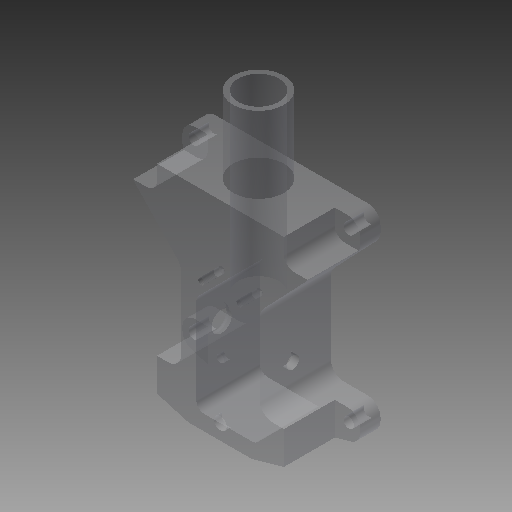
# Autodesk Inventor part: LCD Olfaktometerkammer
Saved by Autodesk Inventor 2018 (Build 220112000, 112)
## iProperties
Created: 2010-08-23
Part Number: LCD Olfaktometerkammer
Document SubType Name: Modeling
Designer: neef
Density: 1 g/cm^3
Material: Generic
Appearance: Polycarbonate - Clear
Author: neef
Autodesk Inventor part; units mm, degrees
ref_plane "YZ Plane" through (0, 0, 0) normal (1, 0, 0) x (0, 1, 0)
ref_plane "XZ Plane" through (0, 0, 0) normal (0, 1, 0) x (-1, 0, 0)
ref_plane "XY Plane" through (0, 0, 0) normal (0, 0, 1) x (1, 0, 0)
sketch "Skizze1" plane through (0, 0, 0) normal (0, 0, 1) x (1, 0, 0)
  line L0 (-3.4427, -24.7647) -> (-3.4427, -50.7647) projected
  line L1 (-3.4427, -50.7647) -> (-23.4427, -50.7647) projected
  line L2 (-23.4427, -50.7647) -> (-23.4427, -24.7647) projected
  line L3 (-23.4427, -24.7647) -> (-3.4427, -24.7647) projected
  circle A0 centre (-43.9427, -51.2647) radius 2.1 projected
  circle A1 centre (17.0573, -51.2647) radius 2.1 projected
  circle A2 centre (17.0573, 14.7353) radius 2.1 projected
  circle A3 centre (-43.9427, 14.7353) radius 2.1 projected
  line L4 (21.5573, 19.2353) -> (21.5573, -55.7647) projected
  line L5 (-48.4427, 19.2353) -> (21.5573, 19.2353) projected
  line L6 (-48.4427, -55.7647) -> (-48.4427, 19.2353) projected
  line L7 (21.5573, -55.7647) -> (-48.4427, -55.7647) projected
  line L8 (-48.4427, 19.2353) -> (21.5573, 19.2353)
  line L9 (21.5573, 19.2353) -> (21.5573, -55.7647)
  line L10 (-48.4427, -55.7647) -> (-48.4427, 19.2353)
  line L11 (0, 37.2353) -> (0, -88.7647) projected
  line L12 (-62.4427, 0) -> (35.5573, 0) projected
  line L13 (-48.4427, -55.7647) -> (-48.4427, -70.7647)
  line L14 (-48.4427, -70.7647) -> (21.5573, -70.7647)
  line L15 (21.5573, -70.7647) -> (21.5573, -55.7647)
  dimension "d9" = 15
  constraints: 12 end point, 3 perpendicular, 2 parallel, 1 horizontal
  measures "d9" distance between parallel lines of L7 L14
extrude "Extrusion1" add sketch "Skizze1" along normal blind 28 contours L0 L1 L2 L3 | A0 | A1 | A2 | A3 | L4 L12 L11 L5 | L4 L7 L11 L12 | L11 L12 L6 L5 | L15 L14 L11 L7 | L11 L7 L6 L12 | L11 L14 L13 L7
sketch "Skizze2" plane through (0, 0, 0) normal (0, 0, -1) x (-1, 0, 0)
  line L0 (-21.5573, -70.7647) -> (-21.5573, 19.2353) projected
  line L1 (0.9427, -19.7647) -> (25.9427, -19.7647)
  line L2 (25.9427, -19.7647) -> (25.9427, -59.7647)
  line L3 (25.9427, -59.7647) -> (0.9427, -59.7647)
  line L4 (0.9427, -59.7647) -> (0.9427, -19.7647)
  line L5 (3.4427, -50.7647) -> (3.4427, -24.7647) projected
  line L6 (48.4427, 19.2353) -> (48.4427, -70.7647) projected
  line L7 (-21.5573, 19.2353) -> (48.4427, 19.2353) projected
  line L8 (-21.5573, -70.7647) -> (-21.5573, 19.2353) projected
  line L9 (3.4427, -24.7647) -> (23.4427, -24.7647) projected
  line L10 (23.4427, -24.7647) -> (23.4427, -50.7647) projected
  line L11 (23.4427, -50.7647) -> (3.4427, -50.7647) projected
  line L12 (48.4427, -70.7647) -> (-21.5573, -70.7647) projected
  point P0 (-21.5573, -55.7647)
  dimension "d2" = 25
  dimension "d3" = 40
  dimension "d5" = 22.5
  dimension "d6" = 5
  constraints: 8 end point, 2 parallel, 1 horizontal, 1 perpendicular
  measures "d2" distance of L2.end L3.end
  measures "d3" distance of L1.end L2.end
  measures "d5" distance between parallel lines of L4 L0
  measures "d6" distance between parallel lines of L9 L1
extrude "Extrusion2" cut sketch "Skizze2" against normal blind 25 contours L1 L2 L3 L4 | L5 L9 L10 L11
sketch "Skizze3" plane through (-48.4427, 19.2353, 0) normal (0, 1, 0) x (1, 0, 0)
  line L0 (0, -28) -> (70, -28) projected
  line L1 (70, 0) -> (70, -28) projected
  circle A0 centre (35, -13) radius 10
  circle A1 centre (35, -13) radius 8
  dimension "d10" = 16
  dimension "d11" = 20
  dimension "d12" = 15
  dimension "d13" = 35
  constraints: 2 centre point, 1 coincident
  measures "d10" diameter of A1
  measures "d11" diameter of A0
  measures "d12" distance from line of L0 A1.centre
  measures "d13" distance from line of L1 A1.centre
extrude "Extrusion3" add sketch "Skizze3" along normal blind 30
sketch "Skizze4" plane through (-13.4427, 19.2353, 13) normal (0, 1, 0) x (1, 0, 0)
  circle A0 centre (0, 0) radius 8 projected
  circle A1 centre (0, 0) radius 8 projected
  circle A2 centre (0, 0) radius 8
  constraints: 1 centre point, 1 coincident, 1 concentric
extrude "Extrusion4" cut sketch "Skizze4" against normal up to surface (39 mm away)
fillet "Rundung1" radius 3 4 edges at (-0.9427, -19.7647, 12.5) (-25.9427, -19.7647, 12.5) (-0.9427, -59.7647, 12.5) (-25.9427, -59.7647, 12.5)
sketch "Skizze5" plane through (0, 0, 28) normal (0, 0, 1) x (1, 0, 0)
  circle A0 centre (-43.9427, 14.7353) radius 2.1 projected
  circle A1 centre (17.0573, 14.7353) radius 2.1 projected
  circle A2 centre (17.0573, -51.2647) radius 2.1 projected
  circle A3 centre (-43.9427, -51.2647) radius 2.1 projected
extrude "Extrusion5" cut sketch "Skizze5" against normal up to surface (28 mm away)
sketch "Skizze6" plane through (0, 0, 25) normal (0, 0, -1) x (-1, 0, 0)
  line L0 (25.9427, -56.7647) -> (25.9427, -22.7647) projected
  line L1 (22.9427, -19.7647) -> (3.9427, -19.7647) projected
  circle A0 centre (13.4427, -34.7647) radius 1.5
  line L2 (3.9427, -59.7647) -> (22.9427, -59.7647) projected
  circle A1 centre (13.4427, -56.7647) radius 2.5
  dimension "d21" = 3
  dimension "d22" = 15
  dimension "d23" = 12.5
  dimension "d58" = 5
  dimension "d59" = 12.5
  dimension "d60" = 3
  constraints: 2 centre point
  measures "d21" diameter of A0
  measures "d22" distance from line of L1 A0.centre
  measures "d23" distance from line of L0 A0.centre
  measures "d58" diameter of A1
  measures "d59" distance from line of L0 A1.centre
  measures "d60" distance from line of L2 A1.centre
extrude "Extrusion6" cut sketch "Skizze6" against normal up to surface (3 mm away)
sketch "Skizze7" plane through (21.5573, -70.7647, 0) normal (1, 0, 0) x (0, 0, -1)
  circle A0 centre (-15, 36) radius 2.45
  line L0 (-25, 37.5) -> (-28, 37.5) projected
  line L1 (-25, 34.5) -> (-28, 34.5) projected
  line L2 (-25, 48) -> (-25, 14) projected
  line L3 (0, 48) -> (-25, 48) projected
  dimension "d26" = 1.5
  dimension "d27" = 4.9
  dimension "d28" = 10
  constraints: 1 centre point
  measures "d26" distance from line of A0.centre L1
  measures "d27" diameter of A0
  measures "d28" distance from line of L2 A0.centre
extrude "Extrusion7" cut sketch "Skizze7" against normal up to surface (70 mm away)
sketch "Skizze8" plane through (0, 0, 0) normal (0, 0, -1) x (-1, 0, 0)
  circle A0 centre (43.9427, -51.2647) radius 2.1 projected
  circle A1 centre (43.9427, 14.7353) radius 2.1 projected
  circle A2 centre (-17.0573, 14.7353) radius 2.1 projected
  circle A3 centre (-17.0573, -51.2647) radius 2.1 projected
  line L0 (0.9427, -56.7647) -> (0.9427, -22.7647) projected
  arc A4 (3.9427, -19.7647) -> (0.9427, -22.7647) centre (3.9427, -22.7647) ccw projected
  line L1 (3.9427, -19.7647) -> (22.9427, -19.7647) projected
  arc A5 (25.9427, -22.7647) -> (22.9427, -19.7647) centre (22.9427, -22.7647) ccw projected
  line L2 (25.9427, -22.7647) -> (25.9427, -56.7647) projected
  arc A6 (22.9427, -59.7647) -> (25.9427, -56.7647) centre (22.9427, -56.7647) ccw projected
  line L3 (22.9427, -59.7647) -> (3.9427, -59.7647) projected
  arc A7 (0.9427, -56.7647) -> (3.9427, -59.7647) centre (3.9427, -56.7647) ccw projected
  line L4 (48.4427, 19.2353) -> (48.4427, -70.7647) projected
  line L5 (-21.5573, 19.2353) -> (48.4427, 19.2353) projected
  line L6 (-21.5573, -70.7647) -> (-21.5573, 19.2353) projected
  line L7 (48.4427, -70.7647) -> (-21.5573, -70.7647) projected
  line L8 (13.4427, -79.9912) -> (13.4427, -69.4061)
  line L9 (48.4427, -70.7647) -> (-21.5573, -70.7647) projected
  line L10 (13.4427, -69.4061) -> (13.4427, 58.2519)
  line L11 (-21.5573, 19.2353) -> (48.4427, 19.2353) projected
  line L12 (13.4427, 19.2353) -> (-16.5573, 19.2353)
  line L13 (-21.5573, 19.2353) -> (-21.5573, 9.7353)
  line L14 (-21.5573, 19.2353) -> (-21.5573, -70.7647) projected
  line L15 (-20.18, 8.2875) -> (-3.4345, -9.3169)
  line L16 (-2.0573, -12.7629) -> (-2.0573, -41.2647)
  line L17 (-7.0573, -46.2647) -> (-16.5573, -46.2647)
  line L18 (-21.5573, 11.7335) -> (-21.5573, 14.2353)
  line L19 (-21.5573, -46.2647) -> (-21.5573, 19.2353)
  line L20 (13.4427, -62.7647) -> (1.6505, -62.7647)
  line L21 (0.2628, -62.5683) -> (-17.9449, -57.3083)
  line L22 (-21.5573, -52.5047) -> (-21.5573, -51.2647)
  arc A8 (-16.5573, 19.2353) -> (-21.5573, 14.2353) centre (-16.5573, 14.2353) ccw
  arc A9 (-21.5573, 11.7335) -> (-20.18, 8.2875) centre (-16.5573, 11.7335) ccw
  arc A10 (-2.0573, -12.7629) -> (-3.4345, -9.3169) centre (-7.0573, -12.7629) ccw
  arc A11 (-7.0573, -46.2647) -> (-2.0573, -41.2647) centre (-7.0573, -41.2647) ccw
  arc A12 (-16.5573, -46.2647) -> (-21.5573, -51.2647) centre (-16.5573, -51.2647) ccw
  arc A13 (-21.5573, -52.5047) -> (-17.9449, -57.3083) centre (-16.5573, -52.5047) ccw
  arc A14 (0.2628, -62.5683) -> (1.6505, -62.7647) centre (1.6505, -57.7647) ccw
  circle A15 centre (43.9427, 14.7353) radius 2.1
  circle A16 centre (43.9427, -51.2647) radius 2.1
  line L23 (48.4427, -70.7647) -> (48.4427, 19.2353)
  line L24 (13.4427, 19.2353) -> (43.4427, 19.2353)
  line L25 (48.4427, 19.2353) -> (48.4427, 9.7353)
  line L26 (47.0655, 8.2875) -> (30.32, -9.3169)
  line L27 (28.9427, -12.7629) -> (28.9427, -41.2647)
  line L28 (33.9427, -46.2647) -> (43.4427, -46.2647)
  line L29 (48.4427, 11.7335) -> (48.4427, 14.2353)
  line L30 (13.4427, -62.7647) -> (25.235, -62.7647)
  line L31 (26.6227, -62.5683) -> (44.8304, -57.3083)
  line L32 (48.4427, -52.5047) -> (48.4427, -51.2647)
  arc A17 (48.4427, 14.2353) -> (43.4427, 19.2353) centre (43.4427, 14.2353) ccw
  arc A18 (47.0655, 8.2875) -> (48.4427, 11.7335) centre (43.4427, 11.7335) ccw
  arc A19 (30.32, -9.3169) -> (28.9427, -12.7629) centre (33.9427, -12.7629) ccw
  arc A20 (28.9427, -41.2647) -> (33.9427, -46.2647) centre (33.9427, -41.2647) ccw
  arc A21 (48.4427, -51.2647) -> (43.4427, -46.2647) centre (43.4427, -51.2647) ccw
  arc A22 (44.8304, -57.3083) -> (48.4427, -52.5047) centre (43.4427, -52.5047) ccw
  arc A23 (25.235, -62.7647) -> (26.6227, -62.5683) centre (25.235, -57.7647) ccw
  point P0 (-2.0573, -10.7647)
  point P1 (0.9427, -62.7647)
  point P2 (-21.5573, -56.2647)
  point P3 (28.9427, -10.7647)
  point P4 (48.4427, -46.2647)
  point P5 (25.9427, -62.7647)
  point P6 (48.4427, -56.2647)
  dimension "d47" = 0
  dimension "d48" = 3
  dimension "d49" = 35
  dimension "d50" = 5
  dimension "d51" = 5
  dimension "d52" = 3
  dimension "d53" = 30
  dimension "d54" = 5
  dimension "d55" = 5
  constraints: 44 end point, 31 symmetric about line, 30 point on line, 28 point on circle, 16 centre point, 14 tangent, 6 equal radius, 6 perpendicular, 2 collinear, 1 midpoint, 1 parallel, 9 other
  measures "d47" distance from line of L0 point (0.943, -62.765)
  measures "d48" distance between parallel lines of L3 L20
  measures "d49" distance between parallel lines of L6 L10
  measures "d50" vertical distance of A3.centre point (-21.557, -56.265)
  measures "d51" distance from line of A3.centre L17
  measures "d52" distance between parallel lines of L0 L16
  measures "d53" distance from line of L5 point (-2.057, -10.765)
  measures "d54" vertical distance of A2.centre L13.end
  measures "d55" radius of A8
extrude "Extrusion8" cut sketch "Skizze8" against normal blind 30 contours L30 A23 L31 A22 L4 L7 L8 L10 | L10 L8 L7 L6 A13 L21 A14 L20 | A8 L6 L5 | L5 L4 A17 | A9 L15 A10 L16 A11 L17 A12 L6 | L4 A21 L28 A20 L27 A19 L26 A18
sketch "Skizze9" plane through (0, 0, 28) normal (0, 0, 1) x (1, 0, 0)
  circle A0 centre (17.0573, -51.2647) radius 2.1 projected
  circle A1 centre (17.0573, 14.7353) radius 2.1 projected
  circle A2 centre (-43.9427, 14.7353) radius 2.1 projected
  circle A3 centre (-43.9427, -51.2647) radius 2.1 projected
  circle A4 centre (17.0573, -51.2647) radius 2.1 projected
  line L0 (-43.4427, 19.2353) -> (16.5573, 19.2353) projected
  line L1 (-48.4427, 11.7335) -> (-48.4427, 14.2353) projected
  arc A5 (-48.4427, 11.7335) -> (-47.0655, 8.2875) centre (-43.4427, 11.7335) ccw projected
  line L2 (-33.9427, -46.2647) -> (-43.4427, -46.2647) projected
  line L3 (-48.4427, -52.5047) -> (-48.4427, -51.2647) projected
  line L4 (21.5573, -51.2647) -> (21.5573, -52.5047) projected
  line L5 (16.5573, -46.2647) -> (7.0573, -46.2647) projected
  arc A6 (20.18, 8.2875) -> (21.5573, 11.7335) centre (16.5573, 11.7335) ccw projected
  line L6 (21.5573, 14.2353) -> (21.5573, 11.7335) projected
  line L7 (16.5573, 19.2353) -> (-43.4427, 19.2353) projected
  line L8 (-38.4427, 19.2353) -> (-38.4427, 13.2353)
  line L9 (-42.4427, 9.2353) -> (-47.7739, 9.2353)
  line L10 (-30.32, -9.3169) -> (-47.0655, 8.2875) projected
  arc A7 (-42.4427, 9.2353) -> (-38.4427, 13.2353) centre (-42.4427, 13.2353) ccw
  line L11 (11.5573, 19.2353) -> (11.5573, 13.2353)
  line L12 (15.5573, 9.2353) -> (20.8884, 9.2353)
  arc A8 (11.5573, 13.2353) -> (15.5573, 9.2353) centre (15.5573, 13.2353) ccw
  line L13 (11.5573, -46.2647) -> (11.5573, -59.1536)
  line L14 (17.9449, -57.3083) -> (-0.2628, -62.5683) projected
  line L15 (-38.4427, -46.2647) -> (-38.4427, -59.1536)
  line L16 (-26.6227, -62.5683) -> (-44.8304, -57.3083) projected
  arc A9 (21.5573, 14.2353) -> (16.5573, 19.2353) centre (16.5573, 14.2353) ccw projected
  arc A10 (-43.4427, 19.2353) -> (-48.4427, 14.2353) centre (-43.4427, 14.2353) ccw projected
  arc A11 (-43.4427, -46.2647) -> (-48.4427, -51.2647) centre (-43.4427, -51.2647) ccw projected
  arc A12 (-48.4427, -52.5047) -> (-44.8304, -57.3083) centre (-43.4427, -52.5047) ccw projected
  line L17 (-0.2628, -62.5683) -> (17.9449, -57.3083) projected
  arc A13 (17.9449, -57.3083) -> (21.5573, -52.5047) centre (16.5573, -52.5047) ccw projected
  arc A14 (21.5573, -51.2647) -> (16.5573, -46.2647) centre (16.5573, -51.2647) ccw projected
  line L18 (-38.4427, 19.2353) -> (-43.4427, 19.2353)
  arc A15 (-43.4427, 19.2353) -> (-48.4427, 14.2353) centre (-43.4427, 14.2353) ccw projected
  line L19 (-48.4427, 14.2353) -> (-48.4427, 11.7335)
  arc A16 (-48.4427, 11.7335) -> (-47.0655, 8.2875) centre (-43.4427, 11.7335) ccw projected
  arc A17 (-43.4427, 19.2353) -> (-48.4427, 14.2353) centre (-43.4427, 14.2353) ccw
  arc A18 (-48.4427, 11.7335) -> (-47.7739, 9.2353) centre (-43.4427, 11.7335) ccw
  arc A19 (21.5573, 14.2353) -> (16.5573, 19.2353) centre (16.5573, 14.2353) ccw
  arc A20 (20.8884, 9.2353) -> (21.5573, 11.7335) centre (16.5573, 11.7335) ccw
  arc A21 (21.5573, -51.2647) -> (16.5573, -46.2647) centre (16.5573, -51.2647) ccw
  arc A22 (17.9449, -57.3083) -> (21.5573, -52.5047) centre (16.5573, -52.5047) ccw
  arc A23 (-43.4427, -46.2647) -> (-48.4427, -51.2647) centre (-43.4427, -51.2647) ccw
  arc A24 (-48.4427, -52.5047) -> (-44.8304, -57.3083) centre (-43.4427, -52.5047) ccw
  line L20 (-38.4427, -46.2647) -> (-43.4427, -46.2647)
  line L21 (-48.4427, -51.2647) -> (-48.4427, -52.5047)
  line L22 (-44.8304, -57.3083) -> (-38.4427, -59.1536)
  line L23 (21.5573, 11.7335) -> (21.5573, 14.2353)
  line L24 (16.5573, 19.2353) -> (11.5573, 19.2353)
  line L25 (11.5573, -46.2647) -> (16.5573, -46.2647)
  line L26 (7.0573, -46.2647) -> (16.5573, -46.2647) projected
  line L27 (16.5573, -46.2647) -> (11.5573, -46.2647)
  line L28 (21.5573, -51.2647) -> (21.5573, -52.5047)
  line L29 (17.9449, -57.3083) -> (11.5573, -59.1536)
  arc A25 (17.9449, -57.3083) -> (21.5573, -52.5047) centre (16.5573, -52.5047) ccw projected
  point P0 (11.5573, 9.2353)
  dimension "d67" = 10
  dimension "d68" = 10
  dimension "d69" = 4
  dimension "d70" = 10
  dimension "d71" = 10
  dimension "d72" = 4
  dimension "d73" = 10
  dimension "d74" = 10
  constraints: 39 tangent, 34 end point, 22 point on circle, 11 collinear, 10 centre point, 8 point on line, 5 perpendicular, 2 concentric, 2 parallel
  measures "d67" distance between parallel lines of L8 L1
  measures "d68" distance between parallel lines of L7 L9
  measures "d69" radius of A7
  measures "d70" distance of L11.start point (11.557, 9.235)
  measures "d71" distance between parallel lines of L6 L11
  measures "d72" radius of A8
  measures "d73" distance between parallel lines of L4 L13
  measures "d74" distance between parallel lines of L15 L3
extrude "Extrusion9" cut sketch "Skizze9" against normal blind 20
sketch "Skizze10" plane through (0, 0, 28) normal (0, 0, 1) x (1, 0, 0)
  circle A0 centre (-5.9427, -12.2647) radius 3 projected
  circle A1 centre (-20.9427, -12.2647) radius 3 projected
  line L0 (-0.9427, -4.7647) -> (-0.9427, -19.7647) projected
  line L1 (-25.9427, -4.7647) -> (-0.9427, -4.7647) projected
  line L2 (-25.9427, -19.7647) -> (-25.9427, -4.7647) projected
  line L3 (-0.9427, -19.7647) -> (-25.9427, -19.7647) projected
  constraints: 2 coincident
hole "Bohrung1" at (-20.9427, -12.2647, 28) at (-5.9427, -12.2647, 28) direction (0, 0, -1) diameter 2.459 depth 8 tip angle 118 thread size "M3x0.5" class "6H" standard "ISO Metric profile"
sketch "Skizze11" plane through (-28.9427, -41.2647, 0) normal (-1, 0, 0) x (0, 0, 1)
  circle A0 centre (15, 6.5) radius 2.45 projected
  circle A1 centre (15, 6.5) radius 4
  dimension "d82" = 8
  constraints: 1 centre point, 1 coincident
  measures "d82" diameter of A1
extrude "Extrusion10" cut sketch "Skizze11" against normal blind 3
sketch "Skizze12" plane through (-28.9427, -41.2647, 0) normal (-1, 0, 0) x (0, 0, 1)
  circle A0 centre (15, 6.5) radius 4 projected
  circle A1 centre (15, 6.5) radius 5
  dimension "d86" = 10
  constraints: 1 centre point, 1 coincident
  measures "d86" diameter of A1
extrude "Extrusion11" cut sketch "Skizze12" against normal blind 1
body "Solid1"
